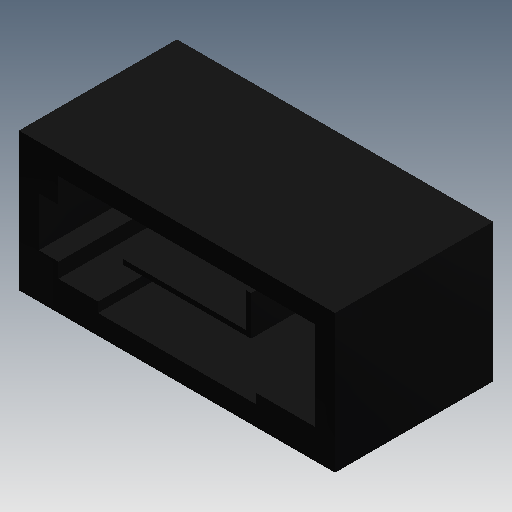
# Autodesk Inventor part: config - j9h2 connector
Saved by Autodesk Inventor 2020 (Build 240152000, 152)
## iProperties
Created: 2005-12-05
Part Number: config - j9h2 connector
Document SubType Name: Modeling
Designer: Simon.Ng@autodesk.com
Stock Number: config - j9h2 connector
Density: 1 g/cm^3
Material: Generic
Mass: 0.516744 g
Surface Area: 9.189 cm^2
Volume: 0.516744 cm^3
Appearance: Glossy - Black
Company: Autodesk Asia Pte. Ltd.
Title: PC Demo
Author: Simon.Ng@autodesk.com
Autodesk Inventor part; units mm, degrees
ref_plane "YZ Plane" through (0, 0, 0) normal (1, 0, 0) x (0, 1, 0)
ref_plane "XZ Plane" through (0, 0, 0) normal (0, 1, 0) x (-1, 0, 0)
ref_plane "XY Plane" through (0, 0, 0) normal (0, 0, 1) x (1, 0, 0)
sketch "Sketch1" plane through (0, 0, 0) normal (0, 0, 1) x (1, 0, 0)
  line L0 (0, 5.6) -> (0, -4.2) projected
  line L1 (-9.6, 0) -> (12.8, 0) projected
  line L2 (-8, 3.5) -> (8, 3.5)
  line L3 (8, 3.5) -> (8, -3.5)
  line L4 (8, -3.5) -> (-8, -3.5)
  line L5 (-8, -3.5) -> (-8, 3.5)
  dimension "d0" = 16
  dimension "d1" = 7
  constraints: 8 end point, 2 parallel, 1 horizontal, 1 perpendicular, 2 other
  measures "d0" distance of L2.start L2.end
  measures "d1" distance of L4.end L2.start
extrude "Extrusion1" add sketch "Sketch1" along normal blind 8
sketch "Sketch2" plane through (0, 0, 8) normal (0, 0, 1) x (1, 0, 0)
  line L0 (8, 3.5) -> (8, -3.5) projected
  line L1 (-6, 2.5) -> (7, 2.5)
  line L2 (7, 2.5) -> (7, -2)
  line L3 (7, -2) -> (-6, -2)
  line L4 (-6, -2) -> (-6, 2.5)
  line L5 (-4, -2) -> (4, -2)
  line L6 (4, -2) -> (4, -2.5)
  line L7 (4, -2.5) -> (-4, -2.5)
  line L8 (-4, -2.5) -> (-4, -2)
  line L9 (-6, 1.25) -> (-7, 1.25)
  line L10 (-7, 1.25) -> (-7, -1.25)
  line L11 (-7, -1.25) -> (-6, -1.25)
  line L12 (-6, -1.25) -> (-6, 1.25)
  line L13 (0, 5.6) -> (0, -4.2) projected
  line L14 (-9.6, 0) -> (12.8, 0) projected
  dimension "d4" = 14
  dimension "d5" = 1
  dimension "d6" = 2.5
  dimension "d7" = 0.5
  dimension "d8" = 5
  dimension "d9" = 1
  dimension "d10" = 8
  constraints: 24 end point, 6 parallel, 3 horizontal, 3 perpendicular, 2 point on line, 3 other
  measures "d4" distance between parallel lines of L2 L10
  measures "d5" distance of L9.start L9.end
  measures "d6" distance of L9.end L10.end
  measures "d7" distance of L7.end L5.start
  measures "d8" distance between parallel lines of L7 L1
  measures "d9" distance between parallel lines of L0 L2
  measures "d10" distance of L6.end L7.end
extrude "Extrusion2" cut sketch "Sketch2" against normal blind 6
sketch "Sketch3" plane through (0, 0, 2) normal (0, 0, 1) x (1, 0, 0)
  line L0 (0, 5.6) -> (0, -4.2) projected
  line L1 (-9.6, 0) -> (12.8, 0) projected
  line L2 (-3.25, 0) -> (3.25, 0)
  line L3 (3.25, 0) -> (3.25, -0.25)
  line L4 (3.25, -0.25) -> (-3.25, -0.25)
  line L5 (-3.25, -0.25) -> (-3.25, 0)
  line L6 (3.25, 0) -> (3, 0)
  line L7 (3, 0) -> (3, 1.75)
  line L8 (3, 1.75) -> (3.25, 1.75)
  line L9 (3.25, 1.75) -> (3.25, 0)
  dimension "d13" = 6.5
  dimension "d14" = 2
  dimension "d15" = 0.25
  dimension "d16" = 0.25
  constraints: 16 end point, 4 parallel, 2 horizontal, 2 perpendicular, 1 point on line, 1 other
  measures "d13" distance of L3.end L4.end
  measures "d14" distance between parallel lines of L4 L8
  measures "d15" distance between parallel lines of L2 L4
  measures "d16" distance between parallel lines of L9 L7
extrude "Extrusion3" add sketch "Sketch3" along normal blind 5.5
sketch "Sketch4" plane through (0, 0, 2) normal (0, 0, 1) x (1, 0, 0)
  line L0 (-3.25, 0) -> (3, 0) projected
  line L1 (3, 0) -> (3, 1.75) projected
  line L2 (2.7, 0) -> (2.3, 0)
  line L3 (2.3, 0) -> (2.3, 0.5)
  line L4 (2.3, 0.5) -> (2.7, 0.5)
  line L5 (2.7, 0.5) -> (2.7, 0)
  dimension "d19" = 0.3
  dimension "d20" = 0.4
  dimension "d21" = 0.5
  constraints: 8 end point, 2 parallel, 1 horizontal, 1 perpendicular, 1 point on line
  measures "d19" distance between parallel lines of L1 L5
  measures "d20" distance of L3.end L4.end
  measures "d21" distance of L2.end L3.end
extrude "Extrusion4" cut sketch "Sketch4" against normal blind 0.5
pattern_linear "Rectangular Pattern1" count 6 spacing 1 along (-1, 0, 0) of "Extrusion4"
equation "\"d15\" = d16"
body "Solid1"
